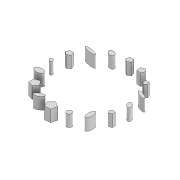
# Autodesk Inventor part: simple_ring1
Saved by Autodesk Inventor 2021 (Build 250183000, 183)
## iProperties
Created: 2022-04-11
Part Number: simple_ring1
Material: Generic
Document SubType Name: Modeling
Designer: Derm
Density: 1 g/cm^3
Appearance: Default
Author: Derm
Autodesk Inventor part; units mm, degrees
ref_plane "YZ Plane" through (0, 0, 0) normal (1, 0, 0) x (0, 1, 0)
ref_plane "XZ Plane" through (0, 0, 0) normal (0, 1, 0) x (-1, 0, 0)
ref_plane "XY Plane" through (0, 0, 0) normal (0, 0, 1) x (1, 0, 0)
sketch "Sketch1" plane through (0, 0, 0) normal (0, 1, 0) x (-1, 0, 0)
  circle A0 centre (0, 0) radius 10000 construction
  circle A1 centre (0, 0) radius 10000 construction
  circle A2 centre (0, 0) radius 10000 construction
  circle A3 centre (0, 0) radius 10000 construction
  circle A4 centre (0, 0) radius 10000 construction
  circle A5 centre (0, 0) radius 10000 construction
  circle A6 centre (0, 0) radius 10000 construction
  circle A7 centre (0, 0) radius 10000 construction
  circle A8 centre (0, 0) radius 10000 construction
  circle A9 centre (0, 0) radius 10000 construction
  circle A10 centre (0, 0) radius 10000 construction
  circle A11 centre (0, 0) radius 10000 construction
  circle A12 centre (0, 0) radius 10000 construction
  circle A13 centre (0, 0) radius 10000 construction
  circle A14 centre (0, 0) radius 10000 construction
  circle A15 centre (0, 0) radius 10000 construction
  ellipse E0 centre (10000, 0) end of major axis (10344.4828, -417.8174) minor radius 397.3786
  ellipse E1 centre (3826.8343, -9238.7953) end of major axis (3005.8343, -8901.6129) minor radius 611.4415
  ellipse E2 centre (3826.8343, 9238.7953) end of major axis (4844.9075, 9810.9569) minor radius 510.0188
  ellipse E3 centre (-9238.7953, -3826.8343) end of major axis (-8019.4501, -4327.616) minor radius 399.5638
  ellipse E4 centre (-3826.8343, 9238.7953) end of major axis (-4072.0909, 8641.6241) minor radius 637.4066
  ellipse E5 centre (-7071.0678, 7071.0678) end of major axis (-6488.3809, 7071.0678) minor radius 1306.202
  ellipse E6 centre (9238.7953, 3826.8343) end of major axis (8014.0127, 3826.8343) minor radius 723.4556
  ellipse E7 centre (7071.0678, -7071.0678) end of major axis (8650.5465, -7358.3167) minor radius 376.7629
  line L0 (5933.0367, 7071.0678) -> (6719.3969, 8153.3997)
  line L1 (6719.3969, 8153.3997) -> (7991.7543, 7739.9857)
  line L2 (7991.7543, 7739.9857) -> (7991.7543, 6402.1499)
  line L3 (7991.7543, 6402.1499) -> (6719.3969, 5988.7359)
  line L4 (6719.3969, 5988.7359) -> (5933.0367, 7071.0678)
  line L5 (9238.7953, -3024.9903) -> (10001.3943, -3579.0509)
  line L6 (10001.3943, -3579.0509) -> (9710.1074, -4475.5397)
  line L7 (9710.1074, -4475.5397) -> (8767.4832, -4475.5397)
  line L8 (8767.4832, -4475.5397) -> (8476.1964, -3579.0509)
  line L9 (8476.1964, -3579.0509) -> (9238.7953, -3024.9903)
  line L10 (-3247.7397, -8631.3844) -> (-3070.2021, -9601.8468)
  line L11 (-3070.2021, -9601.8468) -> (-3938.3045, -10070.5844)
  line L12 (-3938.3045, -10070.5844) -> (-4652.359, -9389.8178)
  line L13 (-4652.359, -9389.8178) -> (-4225.5664, -8500.3433)
  line L14 (-4225.5664, -8500.3433) -> (-3247.7397, -8631.3844)
  line L15 (-750.5685, -9730.2011) -> (24.6556, -9202.7945)
  line L16 (24.6556, -9202.7945) -> (765.8065, -9777.0988)
  line L17 (765.8065, -9777.0988) -> (448.6389, -10659.445)
  line L18 (448.6389, -10659.445) -> (-488.5324, -10630.4606)
  line L19 (-488.5324, -10630.4606) -> (-750.5685, -9730.2011)
  line L20 (-6488.3809, -6844.1933) -> (-6675.2371, -7555.1279)
  line L21 (-6675.2371, -7555.1279) -> (-7409.1179, -7597.1079)
  line L22 (-7409.1179, -7597.1079) -> (-7675.8249, -6912.1184)
  line L23 (-7675.8249, -6912.1184) -> (-7106.7782, -6446.7916)
  line L24 (-7106.7782, -6446.7916) -> (-6488.3809, -6844.1933)
  line L25 (-9006.6059, 3238.6236) -> (-9726.4665, 3424.2419)
  line L26 (-9726.4665, 3424.2419) -> (-9772.3821, 4166.2292)
  line L27 (-9772.3821, 4166.2292) -> (-9080.899, 4439.1843)
  line L28 (-9080.899, 4439.1843) -> (-8607.6232, 3865.8925)
  line L29 (-8607.6232, 3865.8925) -> (-9006.6059, 3238.6236)
  line L30 (110.462, 8737.2386) -> (-1166.8228, 9504.7296)
  line L31 (-1166.8228, 9504.7296) -> (-831.5982, 10956.6675)
  line L32 (-831.5982, 10956.6675) -> (652.8669, 11086.5234)
  line L33 (652.8669, 11086.5234) -> (1235.0921, 9714.8409)
  line L34 (1235.0921, 9714.8409) -> (110.462, 8737.2386)
  ellipse E8 centre (-10000, 0) end of major axis (-9469.8598, -722.4679) minor radius 541.7232
  point P0 (7071.0678, 7071.0678)
  point P1 (0, 10000)
  point P2 (-9238.7953, 3826.8343)
  point P3 (-7071.0678, -7071.0678)
  point P4 (-3826.8343, -9238.7953)
  point P5 (0, -10000)
  point P6 (9238.7953, -3826.8343)
  point P7 (7071.0678, 7071.0678)
  point P8 (9238.7953, -3826.8343)
  point P9 (-3826.8343, -9238.7953)
  point P10 (0, -10000)
  point P11 (-7071.0678, -7071.0678)
  point P12 (-9238.7953, 3826.8343)
  point P13 (0, 10000)
  dimension "d0" = 20000
  dimension "d3" = 360
  constraints: 70 end point, 19 coincident, 6 centre point, 2 horizontal alignment, 2 vertical alignment, 178 other
extrude "Extrusion1" add sketch "Sketch1" along normal mid plane 3000
body "Solid1"
